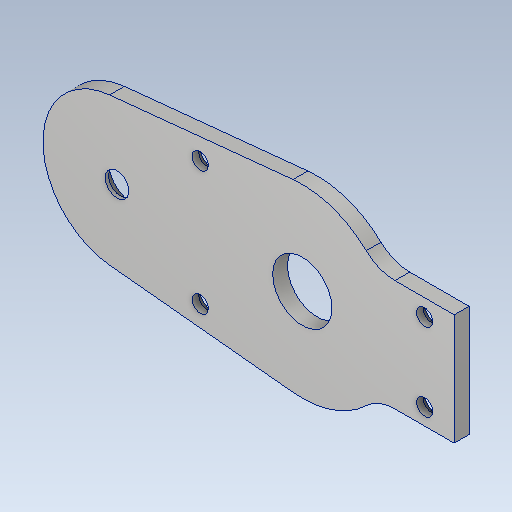
# Autodesk Inventor part: Lower_Arm_v3
Saved by Autodesk Inventor 2021.4 (Build 254397000, 397)
## iProperties
Created: 2020-04-27
Part Number: Lower_Arm_v3
Material: Aluminum 6061
Document SubType Name: Modeling
Designer: Alex
Density: 2.7 g/cm^3
Appearance: Aluminum - Flat
Mass: 5.44663 g
Surface Area: 24.442 cm^2
Volume: 2.01727 cm^3
Flansch_Hole_Dia: 9,750 mm
CounterWeight_Swing_Rad: 25,000 mm
JointFixation_DiaOut: 25,000 mm
LowerArm_Back_DiaOut: 20,000 mm
LowerArm_ShaftFixation_Width: 8,000 mm
ShaftFixation_Width: 15,000 mm
LowerArm_Cover_FixationHole: 14,000 mm
Author: Alex
Autodesk Inventor part; units mm, degrees
ref_plane "YZ Plane" through (0, 0, 0) normal (1, 0, 0) x (0, 1, 0)
ref_plane "XZ Plane" through (0, 0, 0) normal (0, 1, 0) x (-1, 0, 0)
ref_plane "XY Plane" through (0, 0, 0) normal (0, 0, 1) x (1, 0, 0)
sketch "Skizze1" plane through (0, 0, 0) normal (0, 0, 1) x (1, 0, 0)
  line L0 (0, 0) -> (20.5, 0) construction
  circle A0 centre (-25, 0) radius 2.25 construction
  line L1 (-25, 0) -> (0, 0) construction
  line L2 (-26, -9.9499) -> (-1.25, -12.4373)
  line L3 (-1.25, 12.4373) -> (-26, 9.9499)
  arc A1 (-26, 9.9499) -> (-26, -9.9499) centre (-25, 0) ccw
  arc A2 (-1.25, -12.4373) -> (-1.25, 12.4373) centre (0, 0) ccw construction
  circle A3 centre (0, 0) radius 4
  arc A4 (8.6207, 9.0517) -> (12.5, 7.5) centre (12.5, 13.125) ccw
  arc A5 (12.5, -7.5) -> (8.6207, -9.0517) centre (12.5, -13.125) ccw
  line L4 (12.5, 7.5) -> (20.5, 7.5)
  line L5 (20.5, 7.5) -> (20.5, -7.5)
  line L6 (20.5, -7.5) -> (12.5, -7.5)
  line L7 (12.5, -7.5) -> (12.5, 7.5) construction
  arc A6 (-1.25, -12.4373) -> (8.6207, -9.0517) centre (0, 0) ccw
  arc A7 (8.6207, 9.0517) -> (-1.25, 12.4373) centre (0, 0) ccw
  circle A8 centre (-25, 0) radius 4.875 construction
  line L8 (-25, 0) -> (-25, 4.875) construction
  circle A9 centre (0, 0) radius 10.15 construction
  line L9 (0, 0) -> (0, -10.15) construction
  line L10 (16.5, 5.25) -> (16.5, -5.25) construction
  line L11 (16.5, 7.5) -> (16.5, -7.5) construction
  circle A10 centre (-25, 0) radius 10 construction
  line L12 (-25, 0) -> (-13.7735, -8.3646) construction
  line L13 (-13.7735, -8.3646) -> (-14.0535, -11.1505) construction
  line L14 (-25, 0) -> (-13.7735, 8.3646) construction
  line L15 (-13.7735, 8.3646) -> (-14.0535, 11.1505) construction
  point P0 (-12.5, 0)
  point P1 (12.5, 0)
  point P2 (-29.2219, -2.4375)
  point P3 (-20.7781, -2.4375)
  point P4 (0, -10.15)
  point P5 (0, 10.15)
  point P6 (16.5, 0)
  dimension "d127" = 20.3
  dimension "Flansch_Hole_Dia" = 9.75
  dimension "d101" = 0
  dimension "CounterWeight_Swing_Rad" = 25
  dimension "d103" = 4.5
  dimension "d105" = 8
  dimension "d106" = 15
  dimension "LowerArm_ShaftFixation_Width" = 8
  dimension "d118" = 360
  dimension "d130" = 360
  dimension "d132" = 10.5
  dimension "d140" = 12.5
  dimension "LowerArm_Back_DiaOut" = 20
  dimension "d142" = 2.8
  dimension "LowerArm_Cover_FixationHole" = 14
  dimension "d144" = 14
  dimension "d145" = 2.8
  constraints: 34 end point, 14 point on circle, 11 tangent, 8 centre point, 8 coincident, 6 midpoint, 5 perpendicular, 4 point on line, 2 equal radius, 2 horizontal, 2 parallel, 2 vertical alignment, 1 collinear, 1 vertical, 14 other
  measures "d101" distance between parallel lines of L1 L0
  measures "CounterWeight_Swing_Rad" distance of L0.start L1.start
  measures "d103" diameter of A0
  measures "d105" diameter of A3
  measures "d106" distance between parallel lines of L6 L4
  measures "LowerArm_ShaftFixation_Width" distance between parallel lines of L5 L7
  measures "d132" distance of L10.start L10.end
  measures "d140" radius of A2
  measures "LowerArm_Back_DiaOut" diameter of A1
  measures "d142" distance of L12.end L13.end
  measures "LowerArm_Cover_FixationHole" distance of L12.start L12.end
  measures "d144" distance of L12.start L14.end
  measures "d145" distance of L15.start L15.end
extrude "Grundprofil" add sketch "Skizze1" along normal blind 2
hole "Hole10" at (-13.7735, -8.3646, 0) at (-13.7735, 8.3646, 0) direction (0, 0, 1) diameter 2.2 depth 12 tip angle 118 countersink diameter 4.4 countersink angle 90 clearance for "Countersunk Flat Head Screw DIN EN ISO 2009" size "M2" standard "DIN"
hole "Hole11" at (16.5, 5.25, 0) at (16.5, -5.25, 0) direction (0, 0, 1) diameter 2.2 depth 3 tip angle 118 countersink diameter 4.4 countersink angle 90 clearance for "Countersunk Raised Head Screw ISO 2010/7047" size "M2" standard "ISO"
hole "Hole12" at (-25, 0, 0) direction (0, 0, 1) diameter 3.2 depth 12 tip angle 118 countersink diameter 6.3 countersink angle 90 clearance for "Countersunk Flat Head Screw DIN EN ISO 2009" size "M3" standard "DIN"
